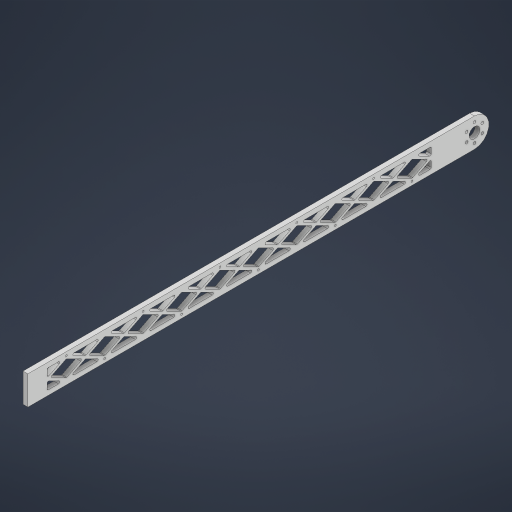
# Autodesk Inventor part: Arm
Saved by Autodesk Inventor 2023 (Build 270158000, 158)
## iProperties
Created: 2023-01-21
Part Number: Arm
Material: Generic
Document SubType Name: Modeling
Designer: Terrence
Density: 1 g/cm^3
Appearance: Default
Author: Terrence
Autodesk Inventor part; units mm, degrees
ref_plane "YZ Plane" through (0, 0, 0) normal (1, 0, 0) x (0, 1, 0)
ref_plane "XZ Plane" through (0, 0, 0) normal (0, 1, 0) x (-1, 0, 0)
ref_plane "XY Plane" through (0, 0, 0) normal (0, 0, 1) x (1, 0, 0)
sketch "Sketch1" plane through (0, 0, 0) normal (1, 0, 0) x (0, 1, 0)
  line L0 (0, 25.4) -> (76.2, 25.4)
  line L1 (76.2, 25.4) -> (76.2, -1193.8)
  line L2 (76.2, -1193.8) -> (0, -1193.8)
  line L3 (0, -1193.8) -> (0, 25.4)
  dimension "d0" = 76.2
  dimension "d1" = 1219.2
  constraints: 8 end point, 2 parallel, 1 horizontal, 1 perpendicular, 1 other
  measures "d0" distance of L1.end L2.end
  measures "d1" distance of L0.end L1.end
extrude "Extrusion1" add sketch "Sketch1" along normal blind 12.7
sketch "Sketch2" plane through (12.7, 0, 0) normal (1, 0, 0) x (0, 0, -1)
  line L0 (1193.8, 76.2) -> (-25.4, 76.2) projected
  line L1 (1155.7, 76.2) -> (1155.7, 0) construction
  line L2 (0, 0) -> (1193.8, 0) projected
  circle A0 centre (1155.7, 38.1) radius 14.2875
  dimension "d5" = 1155.7
  dimension "d24" = 28.575
  constraints: 2 end point, 2 point on line, 1 centre point, 1 midpoint, 1 perpendicular
  measures "d5" distance from line of L2.start L1
  measures "d24" diameter of A0
extrude "Extrusion2" cut sketch "Sketch2" against normal through all
fillet "Fillet1" radius 38.1 2 edges at (6.35, 76.2, -1193.8) (6.35, 0, -1193.8)
sketch "Sketch3" plane through (12.7, 0, 0) normal (1, 0, 0) x (0, 0, -1)
  line L0 (25.4, 63.5) -> (1041.4, 63.5)
  line L1 (1041.4, 63.5) -> (1041.4, 12.7)
  line L2 (1041.4, 12.7) -> (25.4, 12.7)
  line L3 (25.4, 12.7) -> (25.4, 63.5)
  line L4 (0, 0) -> (1155.7, 0) projected
  line L5 (1155.7, 76.2) -> (-25.4, 76.2) projected
  line L6 (-25.4, 76.2) -> (-25.4, 0) projected
  dimension "d9" = 12.7
  dimension "d10" = 12.7
  dimension "d11" = 50.8
  dimension "d12" = 1016
  constraints: 8 end point, 2 parallel, 1 horizontal, 1 perpendicular
  measures "d9" distance between parallel lines of L4 L2
  measures "d10" distance between parallel lines of L5 L0
  measures "d11" distance between parallel lines of L6 L3
  measures "d12" distance of L1.end L2.end
extrude "Extrusion3" cut sketch "Sketch3" against normal through all
sketch "Sketch4" plane through (12.7, 0, 0) normal (1, 0, 0) x (0, 0, -1)
  line L0 (25.4, 63.5) -> (127, 63.5) construction
  line L1 (127, 63.5) -> (127, 12.7) construction
  line L2 (127, 12.7) -> (25.4, 12.7) construction
  line L3 (25.4, 12.7) -> (25.4, 63.5) construction
  line L4 (25.4, 38.1) -> (76.2, 63.5) construction
  line L5 (76.2, 63.5) -> (127, 38.1) construction
  line L6 (127, 38.1) -> (76.2, 12.7) construction
  line L7 (76.2, 12.7) -> (25.4, 38.1) construction
  line L8 (23.9801, 40.9398) -> (74.7801, 66.3398)
  line L9 (74.7801, 66.3398) -> (77.6199, 60.6602)
  line L10 (77.6199, 60.6602) -> (26.8199, 35.2602)
  line L11 (26.8199, 35.2602) -> (23.9801, 40.9398)
  line L12 (23.9801, 40.9398) -> (77.6199, 60.6602) construction
  line L13 (74.7801, 66.3398) -> (26.8199, 35.2602) construction
  line L14 (128.4199, 40.9398) -> (77.6199, 66.3398)
  line L15 (77.6199, 66.3398) -> (74.7801, 60.6602)
  line L16 (74.7801, 60.6602) -> (125.5801, 35.2602)
  line L17 (125.5801, 35.2602) -> (128.4199, 40.9398)
  line L18 (128.4199, 40.9398) -> (74.7801, 60.6602) construction
  line L19 (77.6199, 66.3398) -> (125.5801, 35.2602) construction
  line L20 (23.9801, 35.2602) -> (74.7801, 9.8602)
  line L21 (74.7801, 9.8602) -> (77.6199, 15.5398)
  line L22 (77.6199, 15.5398) -> (26.8199, 40.9398)
  line L23 (26.8199, 40.9398) -> (23.9801, 35.2602)
  line L24 (23.9801, 35.2602) -> (77.6199, 15.5398) construction
  line L25 (74.7801, 9.8602) -> (26.8199, 40.9398) construction
  line L26 (74.7801, 15.5398) -> (125.5801, 40.9398)
  line L27 (125.5801, 40.9398) -> (128.4199, 35.2602)
  line L28 (128.4199, 35.2602) -> (77.6199, 9.8602)
  line L29 (77.6199, 9.8602) -> (74.7801, 15.5398)
  line L30 (74.7801, 15.5398) -> (128.4199, 35.2602) construction
  line L31 (125.5801, 40.9398) -> (77.6199, 9.8602) construction
  point P0 (0, 0)
  point P1 (25.4, 63.5)
  point P2 (50.8, 50.8)
  point P3 (101.6, 50.8)
  point P4 (50.8, 25.4)
  point P5 (101.6, 25.4)
  point P6 (25.4, 38.1)
  point P7 (76.2, 12.7)
  point P8 (76.2, 59.9502)
  point P9 (119.9005, 38.1)
  point P10 (76.2, 16.2498)
  point P11 (32.4995, 38.1)
  point P12 (76.2, 63.5)
  point P13 (127, 38.1)
  dimension "d15" = 101.6
  dimension "d16" = 6.35
  dimension "d17" = 6.35
  constraints: 64 end point, 22 midpoint, 13 parallel, 5 perpendicular, 2 coincident, 2 equal length, 1 horizontal
  measures "d15" distance of L1.end L2.end
  measures "d16" distance of L8.end L9.end
  measures "d17" distance of L15.end L14.end
extrude "Extrusion4" add sketch "Sketch4" against normal up to surface (12.7 mm away) contours L8 L9 L15 L16 L10 L22 L23 L11 | L23 L22 L10 L11 | L11 L10 L22 L26 L29 L21 L20 L23 | L15 L14 L17 L27 L26 L16 L10 L9 | L9 L10 L16 L15 | L26 L16 L17 L27 L28 L29 L21 L22 | L22 L21 L29 L26 | L26 L27 L17 L16
pattern_linear "Rectangular Pattern1" count 10 spacing 101.6 along (0, 0, -1) of "Extrusion4"
fillet "Fillet2" radius 3.175 106 edges at (6.35, 12.7, -25.4) (6.35, 34.5502, -25.4) (6.35, 12.7, -69.1005) (6.35, 16.2498, -76.2) (6.35, 38.1, -32.4995) (6.35, 38.1, -119.9005) (6.35, 59.9502, -76.2) (6.35, 12.7, -170.7005) (6.35, 12.7, -83.2995) (6.35, 12.7, -272.3005) (6.35, 12.7, -184.8995) (6.35, 12.7, -373.9005) (6.35, 12.7, -286.4995) (6.35, 12.7, -475.5005) (6.35, 12.7, -388.0995) (6.35, 12.7, -577.1005) (6.35, 12.7, -489.6995) (6.35, 12.7, -678.7005) (6.35, 12.7, -591.2995) (6.35, 12.7, -780.3005) (6.35, 12.7, -692.8995) (6.35, 12.7, -881.9005) (6.35, 12.7, -794.4995) (6.35, 12.7, -983.5005) (6.35, 12.7, -896.0995) (6.35, 12.7, -1041.4) (6.35, 12.7, -997.6995) (6.35, 34.5502, -1041.4) (6.35, 63.5, -1041.4) (6.35, 41.6498, -1041.4) (6.35, 63.5, -997.6995) (6.35, 63.5, -896.0995) (6.35, 63.5, -983.5005) (6.35, 63.5, -794.4995) (6.35, 63.5, -881.9005) (6.35, 63.5, -692.8995) (6.35, 63.5, -780.3005) (6.35, 63.5, -591.2995) (6.35, 63.5, -678.7005) (6.35, 63.5, -489.6995) (6.35, 63.5, -577.1005) (6.35, 63.5, -388.0995) (6.35, 63.5, -475.5005) (6.35, 63.5, -286.4995) (6.35, 63.5, -373.9005) (6.35, 63.5, -184.8995) (6.35, 63.5, -272.3005) (6.35, 63.5, -83.2995) (6.35, 63.5, -170.7005) (6.35, 41.6498, -127) (6.35, 34.5502, -127) (6.35, 41.6498, -25.4) (6.35, 63.5, -25.4) (6.35, 63.5, -69.1005) (6.35, 41.6498, -228.6) (6.35, 34.5502, -228.6) (6.35, 59.9502, -177.8) (6.35, 38.1, -221.5005) (6.35, 38.1, -134.0995) (6.35, 16.2498, -177.8) (6.35, 34.5502, -330.2) (6.35, 34.5502, -431.8) (6.35, 34.5502, -533.4) (6.35, 34.5502, -635) (6.35, 34.5502, -736.6) (6.35, 34.5502, -838.2) (6.35, 34.5502, -939.8) (6.35, 41.6498, -939.8) (6.35, 41.6498, -838.2) (6.35, 41.6498, -736.6) (6.35, 41.6498, -635) (6.35, 41.6498, -533.4) (6.35, 41.6498, -431.8) (6.35, 41.6498, -330.2) (6.35, 59.9502, -279.4) (6.35, 38.1, -323.1005) (6.35, 38.1, -235.6995) (6.35, 16.2498, -279.4) (6.35, 59.9502, -381) (6.35, 38.1, -424.7005) (6.35, 38.1, -337.2995) (6.35, 16.2498, -381) (6.35, 59.9502, -482.6) (6.35, 38.1, -526.3005) (6.35, 38.1, -438.8995) (6.35, 16.2498, -482.6) (6.35, 59.9502, -584.2) (6.35, 38.1, -627.9005) (6.35, 38.1, -540.4995) (6.35, 16.2498, -584.2) (6.35, 59.9502, -685.8) (6.35, 38.1, -729.5005) (6.35, 38.1, -642.0995) (6.35, 16.2498, -685.8) (6.35, 59.9502, -787.4) (6.35, 38.1, -831.1005) (6.35, 38.1, -743.6995) (6.35, 16.2498, -787.4) (6.35, 59.9502, -889) (6.35, 38.1, -932.7005) (6.35, 38.1, -845.2995) (6.35, 16.2498, -889) (6.35, 59.9502, -990.6) (6.35, 38.1, -1034.3005) (6.35, 38.1, -946.8995) (6.35, 16.2498, -990.6)
sketch "Sketch5" plane through (12.7, 0, 0) normal (1, 0, 0) x (0, 0, -1)
  circle A0 centre (1155.7, 38.1) radius 14.2875 projected
  line L0 (1155.7, 38.1) -> (1155.7, 61.9252) construction
  circle A1 centre (1155.7, 61.9252) radius 3.6233
  point P0 (0, 0)
  dimension "d32" = 23.8252
  constraints: 2 end point, 1 centre point, 1 coincident, 1 vertical
  measures "d32" distance of L0.start L0.end
extrude "Extrusion5" cut sketch "Sketch5" against normal through all contours A1
pattern_circular "Circular Pattern1" count 6 over 360 about axis through (12.7, 38.1, -1155.7) along (-1, 0, 0) of "Extrusion5"
sketch "Sketch6" plane through (12.7, 0, 0) normal (1, 0, 0) x (0, 0, -1)
  circle A0 centre (76.2, 66.675) radius 2.54
  arc A1 (77.6199, 59.2403) -> (74.7801, 59.2403) centre (76.2, 56.4005) ccw projected
  line L0 (76.2, 59.5755) -> (76.2, 76.2) construction
  line L1 (1155.7, 76.2) -> (-25.4, 76.2) projected
  line L2 (76.2, 56.4005) -> (76.2, 58.6744) construction
  circle A2 centre (177.8, 9.525) radius 2.54
  arc A3 (176.3801, 16.9597) -> (179.2199, 16.9597) centre (177.8, 19.7995) ccw projected
  line L3 (177.8, 19.7995) -> (177.8, 16.6245)
  line L4 (0, 0) -> (1155.7, 0) projected
  dimension "d33" = 9.525
  dimension "d34" = 5.08
  dimension "d35" = 9.525
  dimension "d36" = 5.08
  constraints: 6 end point, 3 point on line, 3 vertical, 2 centre point, 2 point on circle, 1 collinear
  measures "d33" distance of L0.end A0.centre
  measures "d34" diameter of A0
  measures "d35" distance from line of L4 A2.centre
  measures "d36" diameter of A2
extrude "Extrusion6" cut sketch "Sketch6" against normal blind 25.4
pattern_linear "Rectangular Pattern2" count 5 spacing -203.2 along (0, 0, 1) of "Extrusion6"
body "Solid1"
